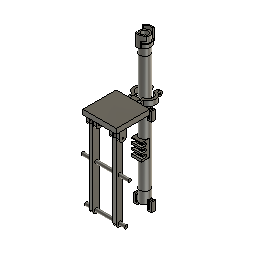
ME270_Project_Assembly (Autodesk Fusion 360 design; units mm, degrees)
Autodesk Fusion 360 part; units mm, degrees
sketch "草图1" plane through (0, 0, 0) normal (0, 0, 1) x (1, 0, 0) in component "Component'"
  circle A0 centre (0, 0) radius 30
  dimension "d1" = 60
  constraint coincident A0.centre origin
  measures "d1" diameter of A0
extrude "拉伸1" add sketch "草图1" along normal blind 200 makes body 1 in component "Component'"
sketch "草图2" plane through (0, 0, 0) normal (0, 0, -1) x (1, 0, 0) in component "Component'"
  circle A0 centre (0, 0) radius 30
  circle A1 centre (0, 0) radius 53
  line L0 (-51.3809, 13) -> (51.3809, 13)
  line L1 (51.3809, -13) -> (-51.3809, -13)
  line L2 (1.75, 0) -> (22.5, 0)
  dimension "d4" = 106
  dimension "d5" = 26
  constraint concentric A0 A1
  constraint coincident A1 L0.start
  constraint coincident A1 L0.end
  constraint horizontal L0
  constraint coincident A1 L1.start
  constraint coincident A1 L1.end
  constraint parallel L0 L1
  constraint symmetric L0 L1 L2
  measures "d4" diameter of A1
  measures "d5" distance of L0 L1
extrude "拉伸2" add sketch "草图2" along normal blind 30 and the other way blind 25 contours A0 A1 L0 L1 | A0 A1 L0 L1 bodies 1 in component "Component'"
ref_plane "工作平面1" through (40.8536, 0, -20) normal (0, 0, -1) x (1, 0, 0) in component "Component'"
sketch "草图3" plane through (39.4089, 0, -20) normal (0, 0, -1) x (1, 0, 0) in component "Component'"
  circle A0 centre (-39.4089, 0) radius 30
  circle A1 centre (-39.4089, 0) radius 44.45
  circle A2 centre (-39.4089, 0) radius 36.1
  arc A3 (-90.7898, 13) -> (-90.7898, -13) centre (-39.4089, 0) ccw
  line L0 (-90.7898, 13) -> (-66.4459, 13)
  arc A4 (-66.4459, 13) -> (-66.4459, -13) centre (-39.4089, 0) ccw
  line L1 (-66.4459, -13) -> (-90.7898, -13)
  arc A5 (11.972, -13) -> (11.972, 13) centre (-39.4089, 0) ccw
  line L2 (11.972, -13) -> (-12.3719, -13)
  arc A6 (-12.3719, -13) -> (-12.3719, 13) centre (-39.4089, 0) ccw
  line L3 (-12.3719, 13) -> (11.972, 13)
  line L4 (-12.3719, 13) -> (11.972, 13)
  point P0 (3.0508, 13)
  point P1 (-5.7309, 13)
  point P2 (3.0976, -13)
  point P3 (-5.7309, -13)
  point P4 (-73.0869, 13)
  point P5 (-81.9154, 13)
  point P6 (-73.0869, -13)
  point P7 (-81.9154, -13)
  dimension "d11" = 88.9
  dimension "d12" = 72.2
  constraint concentric A0 A1
  constraint concentric A1 A2
  constraint coincident L3 P0
  constraint coincident L3 P1
  constraint coincident A2 P1
  constraint coincident L2 P2
  constraint coincident A1 P2
  constraint coincident L2 P3
  constraint coincident A2 P3
  constraint coincident A2 P4
  constraint coincident L0 P4
  constraint coincident A1 P5
  constraint coincident L0 P5
  constraint coincident A2 P6
  constraint coincident L1 P6
  constraint coincident A1 P7
  constraint coincident L1 P7
  measures "d11" diameter of A1
  measures "d12" diameter of A2
sketch "草图4" plane through (0, 0, -30) normal (0, 0, -1) x (1, 0, 0) in component "Component'"
  arc A0 (-51.3809, 13) -> (-51.3809, -13) centre (0, 0) ccw
  line L0 (-51.3809, -13) -> (-27.037, -13)
  arc A1 (-27.037, 13) -> (-27.037, -13) centre (0, 0) ccw
  line L1 (-27.037, 13) -> (-51.3809, 13)
  circle A2 centre (0, 0) radius 44.45
  circle A3 centre (0, 0) radius 36.1
  line L2 (-51.3809, 13) -> (-27.037, 13)
  line L3 (-27.037, -13) -> (-51.3809, -13)
  line L4 (27.037, 13) -> (51.3809, 13)
  line L5 (51.3809, -13) -> (27.037, -13)
extrude "拉伸3" cut sketch "草图4" against normal blind 45 contours L0 L1 A2 A3 L2 L3 | A2 A3 L4 L5 bodies 1 in component "Component'"
extrude "拉伸4" add sketch "草图3" along normal blind 10 contours A1 A2 L2 L3 L4 | A1 A2 L0 L1 bodies 1 in component "Component'"
sketch "草图1 (2)" plane through (0, 0, 0) normal (0, 0, -1) x (1, 0, 0) in component "Component''"
  arc A0 (-27.037, 13) -> (-27.037, -13) centre (0, 0) ccw
  arc A1 (-27.037, -13) -> (27.037, -13) centre (0, 0) ccw
  arc A2 (27.037, -13) -> (27.037, 13) centre (0, 0) ccw
  arc A3 (27.037, 13) -> (-27.037, 13) centre (0, 0) ccw
  circle A4 centre (0, 0) radius 30
  constraint coincident A0.centre A1.centre
extrude "拉伸1'" add sketch "草图1 (2)" along normal blind 400 separate body makes body 2 in component "Component''"
ref_plane "工作平面2" through (0, 0, -45) normal (0, 0, -1) x (-1, 0, 0) in component "Component''"
sketch "草图4 (2)" plane through (0, 0, -45) normal (0, 0, -1) x (1, 0, 0) in component "Component''"
  circle A0 centre (0, 0) radius 36.27
  circle A1 centre (0, 0) radius 44.41
  line L0 (15, 41.8001) -> (15, -41.8001)
  line L1 (-15, -41.8001) -> (-15, 41.8001)
  line L2 (0, -1.75) -> (0, -22.5)
  dimension "d21" = 72.54
  dimension "d22" = 88.82
  dimension "d23" = 30
  constraint coincident A0.centre A1.centre
  constraint coincident A1 L0.start
  constraint coincident A1 L0.end
  constraint vertical L0
  constraint coincident A1 L1.start
  constraint coincident A1 L1.end
  constraint parallel L0 L1
  constraint symmetric L0 L1 L2
  measures "d21" diameter of A0
  measures "d22" diameter of A1
  measures "d23" distance of L0 L1
extrude "拉伸2'" add sketch "草图4 (2)" against normal blind 60 separate body contours A0 A1 L0 L1 | A0 A1 L0 L1 makes body 3 at (13.4193, 33.6962, -5) makes body 4 at (-11.8085, -34.2939, -25) in component "Component''"
sketch "草图5" plane through (0, 0, -45) normal (0, 0, -1) x (1, 0, 0) in component "Component''"
  arc A0 (-15, -41.8001) -> (15, -41.8001) centre (0, 0) ccw
  line L0 (15, -41.8001) -> (15, -33.0229)
  arc A1 (-15, -33.0229) -> (15, -33.0229) centre (0, 0) ccw
  line L1 (-15, -33.0229) -> (-15, -41.8001)
  arc A2 (15, 41.8001) -> (-15, 41.8001) centre (0, 0) ccw
  line L2 (-15, 41.8001) -> (-15, 33.0229)
  arc A3 (15, 33.0229) -> (-15, 33.0229) centre (0, 0) ccw
  line L3 (15, 33.0229) -> (15, 41.8001)
  circle A4 centre (0, 0) radius 36.27
  circle A5 centre (0, 0) radius 30
  dimension "d26" = 72.54
  constraint coincident A0.centre A1.centre
  measures "d26" diameter of A4
extrude "拉伸3'" add sketch "草图5" against normal blind 10 contours A1 A3 A4 bodies 2 3 4 in component "Component''"
extrude "拉伸4'" add 1 faces at (10.1597, 35.2436, -45) along direction (0, 0, -1) blind 10 on bodies 2 bodies 2 in component "Component''"
sketch "草图6" plane through (0, 0, 15) normal (0, 0, 1) x (-1, 0, 0) in component "Component''"
  arc A0 (-15, -41.8001) -> (15, -41.8001) centre (0, 0) ccw
  line L0 (15, -41.8001) -> (15, -33.0229)
  arc A1 (-15, -33.0229) -> (15, -33.0229) centre (0, 0) ccw
  line L1 (-15, -33.0229) -> (-15, -41.8001)
  circle A2 centre (0, 0) radius 36.27
  circle A3 centre (0, 0) radius 44.41
  line L2 (0, 0) -> (36.1229, -25.8338)
  line L3 (0, 0) -> (15, -33.0229)
  line L4 (0, 0) -> (-15, 33.0229)
  line L5 (0, 0) -> (-29.5018, 21.0987)
  line L6 (-29.5018, 21.0987) -> (-36.1229, 25.8338)
  line L7 (-15, 33.0229) -> (-15, 41.8001)
  line L8 (15, -33.0229) -> (15, -41.8001)
  dimension "d31" = 72.54
  dimension "d32" = 88.82
  dimension "d33" = 30
  dimension "d34" = 30
  constraint coincident A0.centre A1.centre
  constraint coincident A3 L2.end
  constraint coincident L0.end A1.end
  constraint coincident A2 L4.end
  constraint parallel L3 L4
  constraint coincident A2 L5.end
  constraint coincident A3 L6.end
  constraint parallel L5 L6
  constraint coincident A3 L7.end
  constraint vertical L7
  constraint coincident A0.end L0.start
  measures "d31" diameter of A2
  measures "d32" diameter of A3
  measures "d33" angle of L2 L3
  measures "d34" angle of L4 L5
extrude "拉伸5" add sketch "草图6" against normal blind 30 contours L0 A2 A3 L2 L8 | A2 A3 L6 L7 bodies 2 in component "Component''"
sketch "草图5 (2)" plane through (0, 0, 200) normal (0, 0, 1) x (-1, 0, 0) in component "Component'"
  circle A0 centre (0, 0) radius 30
  circle A1 centre (0, 0) radius 20
  dimension "d37" = 40
  constraint coincident A0.centre A1.centre
  measures "d37" diameter of A1
extrude "拉伸5'" cut sketch "草图5 (2)" against normal through all contours A1 bodies 1 in component "Component'"
extrude "拉伸6" cut sketch "草图5 (2)" against normal through all contours A1 bodies 2 in component "Component''"
extrude "拉伸6'" cut 1 faces at (-26.5314, 0, 200) along direction (0, 0, -1) blind 130 on bodies 1 bodies 1 in component "Component'"
extrude "拉伸7" cut 1 faces at (-25.2728, -7.9794, -400) along direction (0, 0, 1) blind 300 on bodies 2 bodies 2 in component "Component''"
sketch "草图1 (3)" plane through (0, 0, 25) normal (0, 0, 1) x (-1, 0, 0)
  arc A0 (51.3809, -13) -> (51.3809, 13) centre (0, 0) ccw
  line L0 (51.3809, 13) -> (27.037, 13)
  arc A1 (27.037, -13) -> (27.037, 13) centre (0, 0) ccw
  line L1 (27.037, -13) -> (51.3809, -13)
  arc A2 (42.5065, -13) -> (42.5065, 13) centre (0, 0) ccw
  line L2 (42.5065, -13) -> (33.678, -13)
  arc A3 (33.678, -13) -> (33.678, 13) centre (0, 0) ccw
  line L3 (33.678, 13) -> (42.5065, 13)
  line L4 (-33.678, -13) -> (-42.5065, -13)
  arc A4 (-42.5065, 13) -> (-42.5065, -13) centre (0, 0) ccw
  line L5 (-42.5065, 13) -> (-33.678, 13)
  arc A5 (-33.678, 13) -> (-33.678, -13) centre (0, 0) ccw
extrude "拉伸7'" cut sketch "草图1 (3)" against normal blind 10 contours L0 L1 A2 L2 A3 L3 | L4 A4 L5 A5 bodies 1 in component "Component'"
sketch "Sketch1" plane through (0, 0, 70) normal (0, 0, 1) x (-1, 0, 0) in component "Component'''"
  circle A0 centre (0, 0) radius 20
  circle A1 centre (0, 0) radius 30
sketch "Sketch2" plane through (0, 0, 200) normal (0, 0, -1) x (1, 0, 0) in component "Component'''"
  circle A0 centre (0, 0) radius 20
  circle A1 centre (0, 0) radius 30
extrude "Extrude2" add sketch "Sketch1" along normal up to surface (230 mm away) separate body makes body 5 in component "Component'''"
ref_plane "WorkPlane1" through (0, 0, -80) normal (0, 0, 1) x (1, 0, 0) in component "Component''''"
sketch "Sketch1 (2)" plane through (0, 0, -80) normal (0, 0, 1) x (1, 0, 0) in component "Component''''"
  circle A0 centre (0, 0) radius 30
  circle A1 centre (0, 0) radius 45
  line L0 (0, 45) -> (0, 70)
  line L1 (0, 70) -> (15, 70)
  line L2 (15, 70) -> (15, 42.4264)
  line L3 (0, 70) -> (-15, 70)
  line L4 (-15, 70) -> (-15, 42.4264)
  line L5 (0, -45) -> (0, -70)
  line L6 (0, -70) -> (15, -70)
  line L7 (15, -70) -> (15, -42.4264)
  line L8 (0, -70) -> (-15, -70)
  line L9 (-15, -70) -> (-15, -42.4264)
  line L10 (0, 45) -> (0, 30)
  line L11 (0, -45) -> (0, -30)
  dimension "d84" = 90
  dimension "d85" = 25
  dimension "d86" = 15
  dimension "d87" = 15
  dimension "d88" = 25
  dimension "d89" = 15
  constraint concentric A0 A1
  constraint coincident A1 L0.start
  constraint vertical L0
  constraint perpendicular L0 L1
  constraint coincident A1 L2.end
  constraint perpendicular L1 L2
  constraint perpendicular L0 L3
  constraint coincident A1 L4.end
  constraint perpendicular L3 L4
  constraint coincident A1 L5.start
  constraint parallel L2 L5
  constraint perpendicular L5 L6
  constraint coincident A1 L7.end
  constraint perpendicular L6 L7
  constraint perpendicular L5 L8
  constraint coincident A1 L9.end
  constraint perpendicular L8 L9
  constraint coincident A0 L10.end
  constraint parallel L0 L10
  constraint coincident A0 L11.end
  constraint parallel L5 L11
  measures "d84" diameter of A1
  measures "d85" distance of L5.start L5.end
  measures "d86" distance of L5.end L6.end
  measures "d87" distance of L0.end L1.end
  measures "d88" distance of L0.start L0.end
  measures "d89" distance of L5.end L8.end
extrude "Extrude1" add sketch "Sketch1 (2)" against normal blind 30 separate body contours A0 A1 L10 L11 | A1 L0 L1 L2 | A1 L5 L6 L7 picked at (16.0357, 36.5668) makes body 6 in component "Component''''"
ref_plane "WorkPlane1" through (0, 0, -100) normal (0, 0, 1) x (1, 0, 0) in component "Component'''''"
sketch "Sketch1 (3)" plane through (0, 0, -100) normal (0, 0, 1) x (1, 0, 0) in component "Component'''''"
  circle A0 centre (0, 0) radius 30
  line L0 (20, -70) -> (35, -70)
  line L1 (35, -70) -> (35, -42.4264)
  arc A1 (35, -42.4264) -> (35, 42.4264) centre (20, 0) ccw
  line L2 (35, 42.4264) -> (35, 70)
  line L3 (35, 70) -> (20, 70)
  line L4 (20, 70) -> (20, 30)
  arc A2 (20, -30) -> (20, 30) centre (20, 0) ccw
  line L5 (20, -30) -> (20, -70)
  line L6 (-20, 70) -> (-35, 70)
  line L7 (-35, 70) -> (-35, 42.4264)
  arc A3 (-35, 42.4264) -> (-35, -42.4264) centre (-20, 0) ccw
  line L8 (-35, -42.4264) -> (-35, -70)
  line L9 (-35, -70) -> (-20, -70)
  line L10 (-20, -70) -> (-20, -30)
  arc A4 (-20, 30) -> (-20, -30) centre (-20, 0) ccw
  line L11 (-20, 30) -> (-20, 70)
  line L12 (-20, -30) -> (0, -30)
  line L13 (20, -30) -> (0, -30)
  line L14 (-20, -70) -> (20, -70)
  constraint coincident L10.end A4.end
  constraint coincident A0 L12.end
  constraint tangent A0 L12
  constraint coincident A2.start L5.start
  constraint coincident L9.end L10.start
  constraint coincident L0.start L5.end
extrude "Extrude1'" add sketch "Sketch1 (3)" along normal up to surface (20 mm away) separate body contours L5 L10 L12 L13 L14 makes body 7 in component "Component'''''"
extrude "Extrude2'" add 1 faces at (0, -56.6667, -100) along direction (0, 0, -1) up to surface (10 mm away) on bodies 7 bodies 7 in component "Component'''''"
sketch "Sketch1 (4)" plane through (0, -70, 0) normal (0, -1, 0) x (1, 0, 0) in component "Component''''''"
  line L0 (35, -80) -> (20, -80)
  line L1 (20, -80) -> (20, -110)
  line L2 (20, -110) -> (35, -110)
  line L3 (35, -110) -> (35, -80)
  line L4 (0, -110) -> (0, -80)
  line L5 (0, -80) -> (100, -80)
  line L6 (100, -80) -> (100, -110)
  line L7 (100, -110) -> (0, -110)
  line L8 (0, -110) -> (-100, -110)
  line L9 (-100, -110) -> (-100, -80)
  line L10 (-100, -80) -> (0, -80)
  dimension "d97" = 100
  dimension "d98" = 100
  constraint vertical L4
  constraint perpendicular L3 L5
  constraint perpendicular L5 L6
  constraint perpendicular L6 L7
  constraint perpendicular L4 L8
  constraint perpendicular L8 L9
  constraint perpendicular L4 L10
  measures "d97" distance of L4.end L5.end
  measures "d98" distance of L4.start L8.end
extrude "Extrude1''" add sketch "Sketch1 (4)" along normal blind 200 separate body makes body 8 in component "Component''''''"
extrude "Extrude1'''" add 1 faces at (-15.2228, -21.7676, 0) faces seen with x (1, 0, 0) y (0, 1, 0) z (0, 0, 1) at (0, 0, -170) along direction (0, 0, -1) blind 400 separate body on bodies 1 makes body 9 in component "Component'''''''"
ref_plane "WorkPlane1" through (0, 0, -300) normal (0, 0, 1) x (1, 0, 0) in component "Component''''''''"
sketch "Sketch1 (5)" plane through (0, 0, -300) normal (0, 0, 1) x (1, 0, 0) in component "Component''''''''"
  circle A0 centre (0, 0) radius 30
  line L0 (30, 0) -> (30, -30)
  line L1 (30, -30) -> (-30, -30)
  line L2 (-30, -30) -> (-30, 0)
  line L3 (-30, -30) -> (-30, -50)
  line L4 (-30, -50) -> (30, -50)
  line L5 (30, -50) -> (30, -30)
  constraint coincident A0 L0.start
  constraint tangent A0 L0
  constraint vertical L0
  constraint perpendicular L0 L1
  constraint coincident A0 L2.end
  constraint tangent A0 L2
  constraint perpendicular L1 L2
  constraint perpendicular L1 L3
  constraint perpendicular L3 L4
  constraint perpendicular L1 L5
extrude "Extrude1''''" add sketch "Sketch1 (5)" against normal blind 100 separate body contours A0 L0 L1 | A0 L1 L2 | L1 L3 L4 L5 makes body 10 in component "Component''''''''"
sketch "Sketch2 (2)" plane through (-30, 0, 0) normal (-1, 0, 0) x (0, -1, 0) in component "Component''''''''"
  line L0 (50, -300) -> (0, -300)
  line L1 (0, -300) -> (0, -400)
  line L2 (0, -400) -> (50, -400)
  line L3 (50, -400) -> (50, -300)
  circle A0 centre (30, -380) radius 10
  circle A1 centre (30, -350) radius 10
  circle A2 centre (30, -320) radius 10
  line L4 (50, -365) -> (27.7009, -370.2679)
  line L5 (50, -385) -> (32.585, -389.6601)
  line L6 (50, -335) -> (27.7009, -340.2679)
  line L7 (50, -355) -> (32.585, -359.6601)
  line L8 (50, -305) -> (27.7009, -310.2679)
  line L9 (50, -325) -> (32.585, -329.6601)
  constraint coincident L3 L4.start
  constraint coincident A0 L4.end
  constraint tangent A0 L4
  constraint coincident L3 L5.start
  constraint coincident A0 L5.end
  constraint tangent A0 L5
  constraint coincident L3 L6.start
  constraint coincident A1 L6.end
  constraint tangent A1 L6
  constraint coincident L3 L7.start
  constraint coincident A1 L7.end
  constraint tangent A1 L7
  constraint coincident L3 L8.start
  constraint coincident A2 L8.end
  constraint tangent A2 L8
  constraint coincident L3 L9.start
  constraint coincident A2 L9.end
  constraint tangent A2 L9
extrude "Extrude2''" cut sketch "Sketch2 (2)" against normal through all contours L3 A2 L8 L9 | A2 | L3 A1 L6 L7 | L3 A0 L4 L5 | A1 | A0 bodies 9 in component "Component'''''''"
extrude "Extrude2'''" cut sketch "Sketch2 (2)" against normal through all contours L3 A2 L8 L9 | A2 | L3 A1 L6 L7 | L3 A0 L4 L5 | A1 | A0 bodies 10 in component "Component''''''''"
sketch "Sketch1 (6)" plane through (100, 0, 0) normal (1, 0, 0) x (0, 1, 0) in component "Component'''''''''"
  line L0 (-70, -110) -> (-70, -80)
  line L1 (-70, -80) -> (-270, -80)
  line L2 (-270, -80) -> (-270, -110)
  line L3 (-270, -110) -> (-70, -110)
  line L4 (-250, -110) -> (-210, -110)
  line L5 (-210, -110) -> (-210, -150)
  line L6 (-210, -150) -> (-250, -150)
  line L7 (-250, -150) -> (-250, -110)
  circle A0 centre (-230, -150) radius 20
  circle A1 centre (-230, -150) radius 5
  dimension "d108" = 40
  dimension "d109" = 40
  dimension "d110" = 10
  constraint horizontal L4
  constraint vertical L5
  constraint horizontal L6
  constraint vertical L7
  constraint coincident L3 L4.start
  constraint midpoint L6 A0.centre
  constraint coincident L5.end A0
  constraint concentric A0 A1
  measures "d108" distance of L4.start L4.end
  measures "d109" distance of L4.start L6.end
  measures "d110" diameter of A1
extrude "Extrude1'''''" add sketch "Sketch1 (6)" against normal blind 20 separate body contours L3 L4 L5 L7 A0 | L6 A0 A1 | L6 A0 A1 makes body 11 in component "Component'''''''''"
sketch "Sketch1 (7)" plane through (-80, 0, 0) normal (1, 0, 0) x (0, 1, 0) in component "Component''''''''''"
  circle A0 centre (-230, -150) radius 5
  arc A1 (-250, -150) -> (-210, -150) centre (-230, -150) ccw
  line L0 (-210, -150) -> (-210, -110)
  line L1 (-210, -110) -> (-250, -110)
  line L2 (-250, -110) -> (-250, -150)
  circle A2 centre (-230, -150) radius 20
  line L3 (-250, -150) -> (-250, -350)
  line L4 (-210, -350) -> (-210, -150)
  circle A3 centre (-230, -350) radius 20
  circle A4 centre (-230, -350) radius 10
  line L5 (-210, -350) -> (-210, -600)
  line L6 (-250, -350) -> (-250, -600)
  circle A5 centre (-230, -600) radius 20
  circle A6 centre (-230, -600) radius 10
  dimension "d113" = 20
  dimension "d135" = 250
  dimension "d136" = 250
  constraint concentric A0 A2
  constraint coincident A1.start L2.end
  constraint tangent A2 L3
  constraint parallel L2 L3
  constraint coincident A1.end L0.start
  constraint tangent A2 L4
  constraint coincident L4.start A3
  constraint concentric A3 A4
  constraint parallel L4 L5
  constraint parallel L3 L6
  constraint coincident L6.end A5
  constraint tangent L6 A5
  constraint concentric A5 A6
  measures "d113" diameter of A4
  measures "d135" distance of L4.start L5.end
  measures "d136" distance of L3.end L6.end
extrude "Extrude1''''''" add sketch "Sketch1 (7)" along normal up to surface (20 mm away) separate body contours A1 A2 | A1 A2 L3 L4 A3 | A3 | A3 L5 L6 A5 | A5 makes body 12 in component "Component''''''''''"
sketch "Sketch1 (8)" plane through (-80, 0, 0) normal (-1, 0, 0) x (0, -1, 0) in component "Component'''''''''''"
  circle A0 centre (230, -150) radius 5
  circle A1 centre (230, -350) radius 10
  line L0 (250, -600) -> (250, -150)
  arc A2 (250, -150) -> (210, -150) centre (230, -150) ccw
  line L1 (210, -150) -> (210, -600)
  circle A3 centre (230, -600) radius 10
  arc A4 (210, -600) -> (250, -600) centre (230, -600) ccw
sketch "Sketch2 (3)" plane through (80, 0, 0) normal (1, 0, 0) x (0, 1, 0) in component "Component'''''''''''"
  arc A0 (-210, -150) -> (-250, -150) centre (-230, -150) ccw
  line L0 (-250, -150) -> (-250, -600)
  line L1 (-210, -600) -> (-210, -150)
  circle A1 centre (-230, -150) radius 5
  circle A2 centre (-230, -350) radius 10
  circle A3 centre (-230, -600) radius 10
  arc A4 (-250, -600) -> (-210, -600) centre (-230, -600) ccw
extrude "Extrude1'''''''" add sketch "Sketch1 (8)" against normal blind 160 separate body contours A1 makes body 13 in component "Component'''''''''''"
extrude "Extrude2''''" add 1 faces at (-80, -228.3914, -355.0901) along direction (-1, 0, 0) blind 60 on bodies 13 bodies 13 in component "Component'''''''''''"
extrude "Extrude3" add sketch "Sketch2 (3)" along normal blind 60 contours A2 bodies 13 in component "Component'''''''''''"
sketch "Sketch1 (9)" plane through (-80, 0, 0) normal (-1, 0, 0) x (0, -1, 0) in component "Component''''''''''''"
  circle A0 centre (230, -150) radius 5
  circle A1 centre (230, -350) radius 10
  line L0 (250, -600) -> (250, -150)
  arc A2 (250, -150) -> (210, -150) centre (230, -150) ccw
  line L1 (210, -150) -> (210, -600)
  circle A3 centre (230, -350) radius 20
  line L2 (210, -600) -> (210, -850)
  line L3 (250, -600) -> (250, -850)
  circle A4 centre (157.4159, -850) radius 92.5841
  circle A5 centre (157.4159, -850) radius 10
  circle A6 centre (230, -600) radius 10
  arc A7 (210, -600) -> (250, -600) centre (230, -600) ccw
  dimension "d124" = 250
  dimension "d125" = 250
  dimension "d126" = 20
  constraint concentric A1 A3
  constraint coincident L1.end L2.start
  constraint parallel L1 L2
  constraint coincident L0.start L3.start
  constraint parallel L0 L3
  constraint coincident L3.end A4
  constraint tangent L3 A4
  constraint concentric A4 A5
  measures "d124" distance of L1.end L2.end
  measures "d125" distance of L0.start L3.end
  measures "d126" diameter of A5
extrude "Extrude1''''''''" add sketch "Sketch1 (9)" along normal blind 20 separate body contours A3 makes body 14 in component "Component''''''''''''"
sketch "Sketch1 (10)" plane through (-80, 0, 0) normal (-1, 0, 0) x (0, -1, 0) in component "Component'''''''''''''"
  circle A0 centre (230, -350) radius 10
  circle A1 centre (230, -150) radius 5
  circle A2 centre (230, -600) radius 10
  line L0 (210, -150) -> (210, -600)
  arc A3 (210, -600) -> (250, -600) centre (230, -600) ccw
  line L1 (250, -600) -> (250, -150)
  arc A4 (250, -150) -> (210, -150) centre (230, -150) ccw
extrude "Extrude1'''''''''" add sketch "Sketch1 (10)" against normal blind 200 separate body contours A2 makes body 15 in component "Component'''''''''''''"
extrude "Extrude2'''''" add 1 faces at (-80, -229.8832, -605.6558) along direction (-1, 0, 0) blind 40 on bodies 15 bodies 15 in component "Component'''''''''''''"
fillet "Fillet1" radius 15 1 edges at (0, -30, -80) on bodies 7 in component "Component'''''"
fillet "Fillet2" radius 15 1 edges at (0, -30, -110) on bodies 7 in component "Component'''''"
sketch "Sketch2 (4)" plane through (20, 0, 0) normal (1, 0, 0) x (0, 1, 0) in component "Component'''''"
  arc A0 (-45, -110) -> (-45, -80) centre (-45, -95) ccw
  line L0 (-45, -80) -> (-70, -80)
  line L1 (-70, -80) -> (-70, -110)
  line L2 (-70, -110) -> (-45, -110)
  line L3 (-70, -95) -> (-30, -95)
  line L4 (-57.5, -80) -> (-57.5, -110)
  circle A1 centre (-57.5, -95) radius 5
  dimension "d145" = 10
  constraint midpoint L1 L3.start
  constraint midpoint A0 L3.end
  constraint midpoint L0 L4.start
  constraint midpoint L2 L4.end
  constraint midpoint L4 A1.centre
  measures "d145" diameter of A1
extrude "Extrude3'" cut sketch "Sketch2 (4)" against normal blind 40 contours L3 L4 A1 | L3 L4 A1 | L3 L4 A1 | L3 L4 A1 bodies 7 in component "Component'''''"
sketch "Sketch2 (5)" plane through (0, 0, 0) normal (-1, 0, 0) x (0, -1, 0) in component "Component''''"
  line L0 (-30, -80) -> (-70, -80)
  line L1 (-70, -80) -> (-70, -110)
  line L2 (-70, -110) -> (-30, -110)
  line L3 (-30, -110) -> (-30, -80)
  circle A0 centre (-57.5, -95) radius 5
extrude "Extrude2''''''" cut sketch "Sketch2 (5)" against normal blind 20 contours A0 bodies 6 in component "Component''''"
sketch "Sketch3" plane through (0, 0, 0) normal (-1, 0, 0) x (0, -1, 0) in component "Component''''"
  line L0 (70, -80) -> (30, -80)
  line L1 (30, -80) -> (30, -110)
  line L2 (30, -110) -> (70, -110)
  line L3 (70, -110) -> (70, -80)
  circle A0 centre (57.5, -95) radius 5
extrude "Extrude3''" cut sketch "Sketch3" against normal blind 20 contours A0 bodies 6 in component "Component''''"
fillet "Fillet1'" radius 15 1 edges at (7.5, -70, -80) on bodies 6 in component "Component''''"
fillet "Fillet2'" radius 15 1 edges at (7.5, -70, -110) on bodies 6 in component "Component''''"
fillet "Fillet3" radius 15 1 edges at (7.5, 70, -80) on bodies 6 in component "Component''''"
fillet "Fillet4" radius 15 1 edges at (7.5, 70, -110) on bodies 6 in component "Component''''"
component "Component'" placed x (1, 0, 0) y (0, 1, 0) z (0, 0, 1) at (0, 0, -170)
component "Component''" placed x (1, 0, 0) y (0, 1, 0) z (0, 0, 1) at (0, 0, 230)
component "Component'''" placed x (1, 0, 0) y (0, 1, 0) z (0, 0, 1) at (0, 0, -170)
component "Component''''" placed x (1, 0, 0) y (0, 1, 0) z (0, 0, 1) at (20, 0, 0)
component "Component''''" placed x (-1, 0, 0) y (0, -1, 0) z (0, 0, 1) at (-20, 0, 0)
component "Component'''''" placed x (1, 0, 0) y (0, 1, 0) z (0, 0, 1) at (0, 0, 0)
component "Component''''''" placed x (1, 0, 0) y (0, 1, 0) z (0, 0, 1) at (0, 0, 0)
component "Component'''''''" placed x (1, 0, 0) y (0, 1, 0) z (0, 0, 1) at (0, 0, 0)
component "Component'''''''''" placed x (1, 0, 0) y (0, 1, 0) z (0, 0, 1) at (0, 0, 0)
component "Component''''''''" placed x (1, 0, 0) y (0, 1, 0) z (0, 0, 1) at (0, 0, 0)
component "Component'''''''''" placed x (1, 0, 0) y (0, 1, 0) z (0, 0, 1) at (-180, 0, 0)
component "Component'''''''''" placed x (1, 0, 0) y (0, 1, 0) z (0, 0, 1) at (-140, 0, 0)
component "Component'''''''''" placed x (1, 0, 0) y (0, 1, 0) z (0, 0, 1) at (-40, 0, 0)
component "Component''''''''''" placed x (1, 0, 0) y (0, 1, 0) z (0, 0, 1) at (0, 0, 0)
component "Component''''''''''" placed x (1, 0, 0) y (0, 1, 0) z (0, 0, 1) at (140, 0, 0)
component "Component'''''''''''" placed x (1, 0, 0) y (0, 1, 0) z (0, 0, 1) at (0, 0, 0)
component "Component'''''''''''''" placed x (1, 0, 0) y (0, 1, 0) z (0, 0, 1) at (0, 0, 0)
component "Component'" placed x (1, 0, 0) y (0, 1, 0) z (0, 0, 1) at (0, 0, -640)
